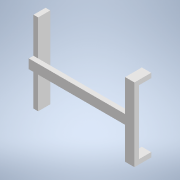
# Autodesk Inventor part: Holder
Saved by Autodesk Inventor 2020 (Build 240168000, 168)
## iProperties
Created: 2020-03-06
Part Number: Holder
Material: Generic
Document SubType Name: Modeling
Designer: Sverrir
Density: 1 g/cm^3
Appearance: Default
Author: Sverrir
Autodesk Inventor part; units mm, degrees
ref_plane "YZ Plane" through (0, 0, 0) normal (1, 0, 0) x (0, 1, 0)
ref_plane "XZ Plane" through (0, 0, 0) normal (0, 1, 0) x (-1, 0, 0)
ref_plane "XY Plane" through (0, 0, 0) normal (0, 0, 1) x (1, 0, 0)
sketch "Sketch1" plane through (0, 0, 0) normal (0, 0, 1) x (1, 0, 0)
  point P0 (0, 0)
sketch "Sketch2" plane through (0, 0, 0) normal (0, 0, 1) x (1, 0, 0)
  line L0 (76.1957, 14.1695) -> (-73.6643, 14.1695) construction
  line L1 (-73.6643, -54.4105) -> (76.1957, -54.4105) construction
  line L2 (34.477, 19.1695) -> (24.477, 19.1695)
  line L3 (24.477, -59.4105) -> (34.477, -59.4105)
  line L4 (34.477, -59.4105) -> (34.477, 19.1695)
  line L5 (24.477, -15.1205) -> (-78.6643, -15.1205)
  line L6 (-78.6643, -15.1205) -> (-78.6643, -25.1205)
  line L7 (-78.6643, -25.1205) -> (24.477, -25.1205)
  line L8 (-73.6643, 14.1695) -> (-73.6643, -54.4105) construction
  line L9 (76.1957, -54.4105) -> (76.1957, 14.1695) construction
  line L10 (76.1957, -20.1205) -> (-73.6643, -20.1205) construction
  line L11 (24.477, 19.1695) -> (24.477, -15.1205)
  line L12 (24.477, -25.1205) -> (24.477, -59.4105)
  line L13 (44.477, -30.2805) -> (44.477, -9.9605) construction
  line L14 (57.177, -30.2805) -> (44.477, -30.2805) construction
  line L15 (57.177, -9.9605) -> (57.177, -30.2805) construction
  line L16 (44.477, -9.9605) -> (57.177, -9.9605) construction
  point P0 (0, 0)
  point P1 (-78.6643, -20.1205)
  dimension "d0" = 5
  dimension "d1" = 5
  dimension "d2" = 5
  dimension "d3" = 10
  dimension "d5" = 10
  dimension "d6" = 10
  constraints: 18 end point, 4 parallel, 3 midpoint, 3 perpendicular, 2 horizontal, 1 collinear, 1 point on line
  measures "d0" distance between parallel lines of L1 L3
  measures "d1" distance between parallel lines of L0 L2
  measures "d2" distance between parallel lines of L8 L6
  measures "d3" distance between parallel lines of L4 L12
  measures "d5" distance between parallel lines of L5 L7
  measures "d6" distance between parallel lines of L4 L13
extrude "Extrusion1" add sketch "Sketch2" along normal blind 5
sketch "Sketch3" plane through (0, 0, 0) normal (0, 0, -1) x (-1, 0, 0)
  line L0 (-76.1957, 14.1695) -> (73.6643, 14.1695) projected
  line L1 (-76.1957, -54.4105) -> (-76.1957, 14.1695) projected
  line L2 (73.6643, -54.4105) -> (-76.1957, -54.4105) projected
  line L3 (73.6643, 14.1695) -> (73.6643, -54.4105) projected
  line L4 (-34.477, -59.4105) -> (-34.477, 19.1695) projected
  line L5 (-24.477, 19.1695) -> (-24.477, -15.1205) projected
  line L6 (-34.477, 19.1695) -> (-24.477, 19.1695)
  line L7 (-24.477, 19.1695) -> (-24.477, 14.1695)
  line L8 (-24.477, 14.1695) -> (-34.477, 14.1695)
  line L9 (-34.477, 14.1695) -> (-34.477, 19.1695)
  line L10 (-24.477, -25.1205) -> (-24.477, -59.4105) projected
  line L11 (-24.477, -59.4105) -> (-34.477, -59.4105)
  line L12 (-34.477, -59.4105) -> (-34.477, -54.4105)
  line L13 (-34.477, -54.4105) -> (-24.477, -54.4105)
  line L14 (-24.477, -54.4105) -> (-24.477, -59.4105)
  line L15 (73.6643, 22.9533) -> (78.6643, 22.9533)
  line L16 (78.6643, 22.9533) -> (78.6643, -64.1223)
  line L17 (78.6643, -64.1223) -> (73.6643, -64.1223)
  line L18 (73.6643, -64.1223) -> (73.6643, 22.9533)
  point P0 (0, 0)
  point P1 (-24.477, -54.4105)
  point P2 (-34.477, -54.4105)
  point P3 (-34.477, 14.1695)
  constraints: 24 end point, 6 parallel, 5 point on line, 3 horizontal, 3 perpendicular
extrude "Extrusion2" add sketch "Sketch3" along normal blind 12.9375 contours L4 L6 L5 L0 | L2 L10 L11 L4 | L18 L15 L16 L17 L3
sketch "Sketch4" plane through (0, 0, 0) normal (0, 0, 1) x (1, 0, 0)
  line L0 (-78.6643, -64.1223) -> (-78.6643, 22.9533) projected
  line L1 (-78.6643, 22.9533) -> (-73.6643, 22.9533)
  line L2 (-73.6643, 22.9533) -> (-73.6643, -64.1223)
  line L3 (-73.6643, -64.1223) -> (-78.6643, -64.1223)
  line L4 (-78.6643, -64.1223) -> (-78.6643, 22.9533)
  point P0 (0, 0)
  constraints: 8 end point, 2 parallel, 1 horizontal, 1 perpendicular
extrude "Extrusion3" add sketch "Sketch4" along normal blind 5
equation "\"d5\" = d3"
body "Solid1"
